Autodesk Fusion 360 part; units mm, degrees
(part 2 of 2)
sketch "Skizze35" plane through (0, 0, 0) normal (0, 0, -1) x (1, 0, 0)
  line L0 (88.062827, 70) -> (88.062827, 67)
  line L1 (88.062827, 67) -> (78.062827, 67)
  line L2 (78.062827, 67) -> (78.062827, 70)
  line L3 (78.062827, 70) -> (33.062827, 70)
  line L4 (33.062827, 70) -> (33.062827, 67)
  line L5 (33.062827, 67) -> (23.062827, 67)
  line L6 (23.062827, 67) -> (23.062827, 70)
  line L7 (23.062827, 70) -> (-21.937173, 70)
  line L8 (-21.937173, 70) -> (-21.937173, 67)
  line L9 (-21.937173, 67) -> (-31.937173, 67)
  line L10 (-31.937173, 67) -> (-31.937173, 70)
  line L11 (-31.937173, 70) -> (-76.937173, 70)
  line L12 (-76.937173, 70) -> (-76.937173, 67)
  line L13 (-76.937173, 67) -> (-86.937173, 67)
  line L14 (-86.937173, 67) -> (-86.937173, 70)
  line L15 (-86.937173, 70) -> (-100, 70)
  line L16 (-100, 70) -> (-100, 60)
  line L17 (-100, 60) -> (-97, 60)
  line L18 (-97, 60) -> (-97, 50)
  line L19 (-97, 50) -> (-100, 50)
  line L20 (-100, 50) -> (-100, 23.333333)
  line L21 (-100, 23.333333) -> (-97, 23.333333)
  line L22 (-97, 23.333333) -> (-97, 13.333333)
  line L23 (-97, 13.333333) -> (-100, 13.333333)
  line L24 (-100, 13.333333) -> (-100, -13.333333)
  line L25 (-100, -13.333333) -> (-97, -13.333333)
  line L26 (-97, -13.333333) -> (-97, -23.333333)
  line L27 (-97, -23.333333) -> (-100, -23.333333)
  line L28 (-100, -23.333333) -> (-100, -50)
  line L29 (-100, -50) -> (-97, -50)
  line L30 (-97, -50) -> (-97, -60)
  line L31 (-97, -60) -> (-100, -60)
  line L32 (-100, -60) -> (-100, -70)
  line L33 (-100, -70) -> (-90.254959, -70)
  line L34 (-90.254959, -70) -> (-90.254959, -67)
  line L35 (-90.254959, -67) -> (-80.254959, -67)
  line L36 (-80.254959, -67) -> (-80.254959, -70)
  line L37 (-80.254959, -70) -> (-33.588293, -70)
  line L38 (-33.588293, -70) -> (-33.588293, -67)
  line L39 (-33.588293, -67) -> (-23.588293, -67)
  line L40 (-23.588293, -67) -> (-23.588293, -70)
  line L41 (-23.588293, -70) -> (23.078374, -70)
  line L42 (23.078374, -70) -> (23.078374, -67)
  line L43 (23.078374, -67) -> (33.078374, -67)
  line L44 (33.078374, -67) -> (33.078374, -70)
  line L45 (33.078374, -70) -> (79.745041, -70)
  line L46 (79.745041, -70) -> (79.745041, -67)
  line L47 (79.745041, -67) -> (89.745041, -67)
  line L48 (89.745041, -67) -> (89.745041, -70)
  line L49 (89.745041, -70) -> (100, -70)
  line L50 (100, -70) -> (100, -61.097561)
  line L51 (100, -61.097561) -> (97, -61.097561)
  line L52 (97, -61.097561) -> (97, -51.097561)
  line L53 (97, -51.097561) -> (100, -51.097561)
  line L54 (100, -51.097561) -> (100, -24.430895)
  line L55 (100, -24.430895) -> (97, -24.430895)
  line L56 (97, -24.430895) -> (97, -14.430895)
  line L57 (97, -14.430895) -> (100, -14.430895)
  line L58 (100, -14.430895) -> (100, 12.235772)
  line L59 (100, 12.235772) -> (97, 12.235772)
  line L60 (97, 12.235772) -> (97, 22.235772)
  line L61 (97, 22.235772) -> (100, 22.235772)
  line L62 (100, 22.235772) -> (100, 48.902439)
  line L63 (100, 48.902439) -> (97, 48.902439)
  line L64 (97, 48.902439) -> (97, 58.902439)
  line L65 (97, 58.902439) -> (100, 58.902439)
  line L66 (100, 58.902439) -> (100, 70)
  line L67 (100, 70) -> (88.062827, 70)
sketch "Skizze36" plane through (0.049959, 70, 31.5) normal (0, 1, 0) x (-1, 0, 0)
  line L0 (79.199998, -28.499999) -> (73.199998, -28.499999)
  line L1 (73.199998, -28.499999) -> (73.199998, -24.499999)
  line L2 (73.199998, -24.499999) -> (79.199998, -24.499999)
  line L3 (79.199998, -24.499999) -> (79.199998, -28.499999)
  dimension "d149" = 6
  dimension "d150" = 4
  constraint horizontal L0
  constraint vertical L1
  constraint horizontal L2
  constraint vertical L3
extrude "Extrusion30" cut sketch "Skizze36" against normal blind 5 bodies 3
sketch "Skizze37" plane through (0, 70, 0) normal (0, 1, 0) x (-1, 0, 0)
named bodies: "Bodenplatte", "Seitenwand Links", "Seitenwand Hinten", "Seitenwand Rechts", "Seitenwand Vorne", "Obereplatte"
